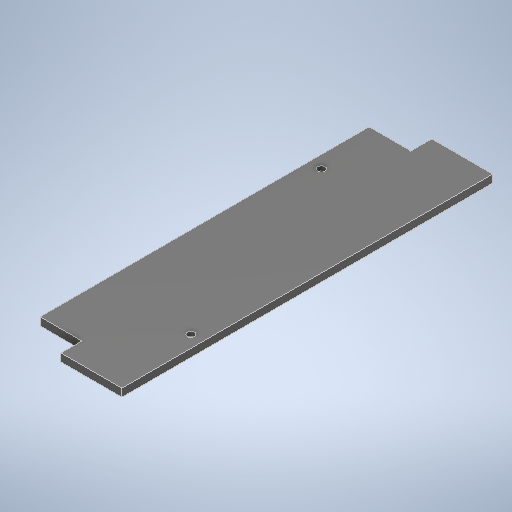
# Autodesk Inventor part: Shelf V1
Saved by Autodesk Inventor 2025 (Build 290162000, 162)
## iProperties
Created: 2025-06-10
Part Number: Shelf V1
Material: Acetal Resin, Black
Document SubType Name: Modeling
Designer: Caleb Fangmeier
Density: 1.425 g/cm^3
Appearance: Smooth - Black
Author: Caleb Fangmeier
Autodesk Inventor part; units mm, degrees
ref_plane "YZ Plane" through (0, 0, 0) normal (1, 0, 0) x (0, 1, 0)
ref_plane "XZ Plane" through (0, 0, 0) normal (0, 1, 0) x (-1, 0, 0)
ref_plane "XY Plane" through (0, 0, 0) normal (0, 0, 1) x (1, 0, 0)
sketch "Sketch1" plane through (0, 0, 0) normal (0, 1, 0) x (-1, 0, 0)
  line L0 (-62.5, -225.7) -> (62.5, -225.7)
  line L1 (62.5, -225.7) -> (62.5, 225.7)
  line L2 (62.5, 225.7) -> (-62.5, 225.7)
  line L3 (-62.5, 225.7) -> (-62.5, -225.7)
  line L4 (-62.5, -225.7) -> (62.5, 225.7) construction
  line L5 (62.5, -225.7) -> (-62.5, 225.7) construction
  point P0 (0, 0)
  dimension "d0" = 451.4
  dimension "d1" = 125
  constraints: 12 end point, 2 midpoint, 2 parallel, 1 horizontal, 1 perpendicular
  measures "d0" distance of L0.end L1.end
  measures "d1" distance of L1.end L2.end
extrude "Extrusion1" add sketch "Sketch1" along normal blind 9.525
sketch "Sketch2" plane through (0, 9.525, 0) normal (0, 1, 0) x (1, 0, 0)
  line L0 (-62.5, 225.7) -> (-62.5, -225.7) projected
  line L1 (-62.5, -225.7) -> (-11.7, -225.7)
  line L2 (-11.7, -225.7) -> (-11.7, -200.3)
  line L3 (-11.7, -200.3) -> (-62.5, -200.3)
  line L4 (-62.5, -200.3) -> (-62.5, -225.7)
  line L5 (-62.5, 225.7) -> (-11.7, 225.7)
  line L6 (-11.7, 225.7) -> (-11.7, 200.3)
  line L7 (-11.7, 200.3) -> (-62.5, 200.3)
  line L8 (-62.5, 200.3) -> (-62.5, 225.7)
  point P0 (0, 0)
  point P1 (-62.5, 200.3)
  dimension "d4" = 25.4
  dimension "d5" = 25.4
  dimension "d6" = 50.8
  dimension "d7" = 50.8
  constraints: 16 end point, 4 parallel, 2 horizontal, 2 perpendicular
  measures "d4" distance of L1.end L2.end
  measures "d5" distance of L5.end L6.end
  measures "d6" distance between parallel lines of L0 L2
  measures "d7" distance of L0.start L5.end
extrude "Extrusion2" cut sketch "Sketch2" against normal through all
sketch "Sketch3" plane through (0, 0, 0) normal (0, 1, 0) x (1, 0, 0)
  line L0 (-62.5, 200.3) -> (-62.5, -200.3) projected
  line L1 (62.5, -225.7) -> (62.5, 225.7) projected
  point P0 (0, 0)
  point P1 (-47.5, 127)
  point P2 (47.7, -127)
  dimension "d10" = 254
  dimension "d11" = 95.2
  dimension "d12" = 127
  dimension "d13" = 15
  dimension "d14" = 14.8
  measures "d10" vertical distance of point (47.7, -127) point (-47.5, 127)
  measures "d11" horizontal distance of point (47.7, -127) point (-47.5, 127)
  measures "d12" vertical distance of point (0, 0) point (-47.5, 127)
  measures "d13" distance from line of L0 point (-47.5, 127)
  measures "d14" distance from line of L1 point (47.7, -127)
hole "Hole1" at (-47.5, 0, -127) at (47.7, 0, 127) direction (0, 1, 0) diameter 9 end through all countersink diameter 17.3 countersink angle 90 clearance for "Flat Head Machine Screw" size "M8" standard "Ansi Metric M Profile"
equation "\"d5\" = d4"
equation "\"d7\" = d6"
equation "\"d12\" = 0.5 * d10"
body "Solid1"
